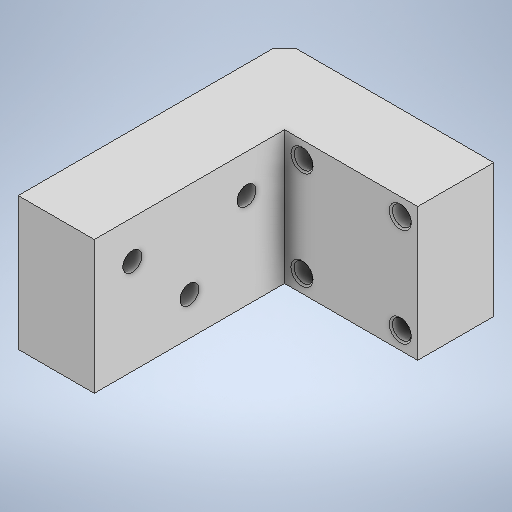
# Autodesk Inventor part: XaxisMotorMount
Saved by Autodesk Inventor 2025.1 (Build 291241000, 241)
## iProperties
Created: 2024-10-09
Part Number: XaxisMotorMount
Material: Generic
Document SubType Name: Modeling
Designer: maxda
Density: 1 g/cm^3
Appearance: Default
Author: maxda
## iProperties of the stored document XaxisMotorMount_3DPrint.ipt
Created: 2024-10-09
Part Number: XaxisMotorMount_3DPrint
Material: Generic
Document SubType Name: Modeling
Designer: maxda
Density: 1 g/cm^3
Appearance: Default
Author: maxda
Autodesk Inventor part; units mm, degrees
ref_plane "YZ Plane" through (0, 0, 0) normal (1, 0, 0) x (0, 1, 0)
ref_plane "XZ Plane" through (0, 0, 0) normal (0, 1, 0) x (-1, 0, 0)
ref_plane "XY Plane" through (0, 0, 0) normal (0, 0, 1) x (1, 0, 0)
sketch "Sketch1" plane through (0, 0, 0) normal (0, 1, 0) x (-1, 0, 0)
  line L0 (0, 0) -> (-42, 0)
  line L1 (-42, 0) -> (-42, -24)
  line L2 (-42, -24) -> (24, -24)
  line L3 (24, -24) -> (24, 60)
  line L4 (24, 60) -> (0, 60)
  line L5 (0, 60) -> (0, 0)
  dimension "d0" = 24
  dimension "d1" = 42
  dimension "d2" = 24
  dimension "d3" = 60
  constraints: 12 end point, 5 perpendicular, 1 horizontal
  measures "d0" distance of L0.end L1.end
  measures "d1" distance of L0.start L0.end
  measures "d2" distance between parallel lines of L5 L3
  measures "d3" distance between parallel lines of L0 L4
extrude "Extrusion1" add sketch "Sketch1" along normal blind 42
sketch "Sketch2" plane through (0, 0, 0) normal (0, 0, 1) x (1, 0, 0)
  circle A0 centre (5.5, 36.5) radius 1.75
  circle A1 centre (36.5, 36.5) radius 1.75
  circle A2 centre (36.5, 5.5) radius 1.75
  circle A3 centre (5.5, 5.5) radius 1.75
  line L0 (42, 0) -> (42, 42) projected
  line L1 (0, 42) -> (42, 42) projected
  point P0 (0, 0)
  dimension "d6" = 3.5
  dimension "d7" = 5.5
  dimension "d8" = 5.5
  dimension "d9" = 31
  dimension "d10" = 31
  constraints: 4 centre point, 3 equal radius, 2 horizontal alignment, 2 vertical alignment
  measures "d6" diameter of A1
  measures "d7" distance from line of L0 A1.centre
  measures "d8" distance from line of L1 A1.centre
  measures "d9" distance of A1.centre A0.centre
  measures "d10" distance of A1.centre A2.centre
extrude "Extrusion2" cut sketch "Sketch2" against normal blind 42
sketch "Sketch3" plane through (0, 0, 60) normal (1, 0, 0) x (0, 0, -1)
  circle A0 centre (12, 30) radius 5
  circle A1 centre (30, 12) radius 5
  circle A2 centre (48, 30) radius 5
  line L0 (12, 30) -> (30, 12) construction
  line L1 (30, 12) -> (48, 30) construction
  line L2 (0, 42) -> (60, 42) construction
  line L3 (0, 0) -> (0, 42) construction
  line L4 (0, 0) -> (60, 0) construction
  line L5 (60, 0) -> (60, 42) construction
  dimension "d13" = 12
  dimension "d14" = 12
  dimension "d15" = 12
  dimension "d16" = 10
  dimension "d17" = 12
  constraints: 4 end point, 3 centre point, 2 equal radius, 1 horizontal alignment, 1 perpendicular
  measures "d13" distance from line of L2 L0.start
  measures "d14" distance from line of L3 L0.start
  measures "d15" distance from line of L4 L0.end
  measures "d16" diameter of A2
  measures "d17" distance from line of L5 L1.end
sketch "Sketch4" plane through (-24, 0, -24) normal (-1, 0, 0) x (0, 0, 1)
  circle A0 centre (54, 12) radius 5 projected
  circle A1 centre (36, 30) radius 5 projected
  circle A2 centre (72, 30) radius 5 projected
  circle A3 centre (54, 12) radius 3
  circle A4 centre (36, 30) radius 3
  circle A5 centre (72, 30) radius 3
  point P0 (24, 0)
  dimension "d20" = 6
  constraints: 3 centre point, 3 coincident, 2 equal radius
  measures "d20" diameter of A3
extrude "Extrusion3" cut sketch "Sketch4" against normal blind 11 contours A0 | A1 | A2 | A3 | A4 | A5
extrude "Extrusion4" cut sketch "Sketch4" against normal blind 32.5 contours A3 | A4 | A5
sketch "Sketch6" plane through (0, 0, 0) normal (0, 0, 1) x (1, 0, 0)
  circle A0 centre (36.5, 5.5) radius 1.75 construction
  circle A1 centre (5.5, 5.5) radius 1.75 construction
  circle A2 centre (5.5, 36.5) radius 1.75 construction
  circle A3 centre (36.5, 36.5) radius 1.75 construction
  circle A4 centre (36.5, 5.5) radius 3
  circle A5 centre (5.5, 5.5) radius 3
  circle A6 centre (5.5, 36.5) radius 3
  circle A7 centre (36.5, 36.5) radius 3
  point P0 (0, 0)
  dimension "d23" = 6
  constraints: 4 centre point, 4 coincident, 3 equal radius
  measures "d23" diameter of A4
extrude "Extrusion5" cut sketch "Sketch6" against normal blind 10
chamfer "Chamfer1" distance 1.25 angle 45 4 edges at (3.75, 5.5, -10) (3.75, 36.5, -10) (34.75, 36.5, -10) (34.75, 5.5, -10)
chamfer "Chamfer2" distance 0.5 angle 45 7 edges at (33.5, 5.5, 0) (2.5, 5.5, 0) (2.5, 36.5, 0) (33.5, 36.5, 0) (-24, 12, 25) (-24, 30, 7) (-24, 30, 43)
chamfer "Chamfer3" distance 3.5 angle 45 1 edges at (-24, 21, -24)
body "Solid1"
